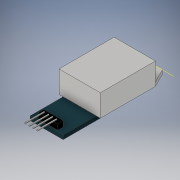
# Autodesk Inventor part: DHT22
Saved by Autodesk Inventor 2017.2 (Build 212223000, 223)
## iProperties
Created: 2017-03-02
Part Number: DHT22
Material: Generic
Document SubType Name: Modeling
Designer: prosp
Density: 1 g/cm^3
Appearance: Default
Author: prosp
Autodesk Inventor part; units mm, degrees
ref_plane "YZ Plane" through (0, 0, 0) normal (1, 0, 0) x (0, 1, 0)
ref_plane "XZ Plane" through (0, 0, 0) normal (0, 1, 0) x (-1, 0, 0)
ref_plane "XY Plane" through (0, 0, 0) normal (0, 0, 1) x (1, 0, 0)
sketch "Sketch1" plane through (0, 0, 0) normal (0, 1, 0) x (-1, 0, 0)
  line L0 (6, 14) -> (6, -14)
  line L1 (6, -14) -> (-6, -14)
  line L2 (-6, -14) -> (-6, 14)
  line L3 (-6, 14) -> (6, 14)
  line L4 (6, 14) -> (-6, -14) construction
  line L5 (6, -14) -> (-6, 14) construction
  line L6 (35.8902, -6.311) -> (20.8902, -6.311)
  line L7 (35.8902, -6.311) -> (35.8902, -26.311)
  line L8 (20.8902, -6.311) -> (20.8902, -26.311)
  line L9 (20.8902, -26.311) -> (23.3902, -31.311)
  line L10 (35.8902, -26.311) -> (33.3902, -31.311)
  line L11 (33.3902, -31.311) -> (23.3902, -31.311)
  point P0 (0, 0)
  dimension "d0" = 28
  dimension "d1" = 12
  dimension "d3" = 15
  dimension "d4" = 20
  dimension "d5" = 20
  constraints: 24 end point, 3 vertical, 2 horizontal, 2 midpoint, 2 parallel, 1 perpendicular, 1 point on line
  measures "d0" distance of L0.start L0.end
  measures "d1" distance of L0.end L1.end
  measures "d3" distance of L6.start L6.end
  measures "d4" distance of L6.start L7.end
  measures "d5" distance of L6.end L8.end
extrude "Extrusion1" add sketch "Sketch1" along normal blind 1.5 contours L0 L1 L2 L3
sketch "Sketch2" plane through (0, 1.5, 0) normal (0, 1, 0) x (1, 0, 0)
  line L0 (-6, -14) -> (6, -14) projected
  line L1 (-7.5, -2) -> (7.5, -2)
  line L2 (7.5, -2) -> (7.5, 18)
  line L3 (-7.5, 18) -> (-7.5, -2)
  line L4 (-7.5, 18) -> (-5, 23)
  line L5 (-5, 23) -> (5, 23)
  line L6 (5, 23) -> (7.5, 18)
  point P0 (0, 0)
  dimension "d14" = 15
  dimension "d15" = 20
  dimension "d16" = 15
  dimension "d19" = 10
  constraints: 12 end point, 2 horizontal, 1 vertical
  measures "d14" distance of L1.start L1.end
  measures "d15" distance of L1.end L2.end
  measures "d16" distance of L2.end L3.start
  measures "d19" distance of L4.end L5.end
extrude "Extrusion2" add sketch "Sketch2" along normal blind 1.5
sketch "Sketch3" plane through (0, 3, 0) normal (0, 1, 0) x (1, 0, 0)
  line L0 (-7.5, 18) -> (-7.5, -2) projected
  line L1 (7.5, -2) -> (7.5, 18) projected
  line L2 (-7.5, -2) -> (7.5, -2)
  line L3 (7.5, -2) -> (7.5, 18)
  line L4 (7.5, 18) -> (-7.5, 18)
  line L5 (-7.5, 18) -> (-7.5, -2)
  point P0 (0, 0)
  constraints: 8 end point, 2 parallel, 1 horizontal, 1 perpendicular
extrude "Extrusion3" add sketch "Sketch3" along normal blind 6.5
sketch "Sketch4" plane through (0, 1.5, 0) normal (0, 1, 0) x (1, 0, 0)
  line L0 (-6, -14) -> (6, -14) projected
  line L1 (-3.5, -13.5) -> (3.5, -13.5)
  line L2 (3.5, -13.5) -> (3.5, -11.5)
  line L3 (3.5, -11.5) -> (-3.5, -11.5)
  line L4 (-3.5, -11.5) -> (-3.5, -13.5)
  point P0 (0, 0)
  dimension "d27" = 7
  dimension "d28" = 2
  dimension "d29" = 7
  constraints: 8 end point, 1 perpendicular
  measures "d27" distance of L1.start L1.end
  measures "d28" distance of L1.end L2.end
  measures "d29" distance of L2.end L3.end
extrude "Extrusion4" add sketch "Sketch4" along normal blind 2
sketch "Sketch5" plane through (0, 3.5, 0) normal (0, 1, 0) x (1, 0, 0)
  point P0 (0, 0)
sketch "Sketch6" plane through (-3.5, 1.5, 13.5) normal (0, 0, 1) x (1, 0, 0)
  line L0 (0, 2) -> (7, 2) projected
  circle A0 centre (2.7375, 2.25) radius 0.25
  circle A1 centre (4.16, 2.25) radius 0.25
  circle A2 centre (5.6263, 2.25) radius 0.25
  circle A3 centre (1.1349, 2.25) radius 0.25
  point P0 (3.5, -1.5)
  dimension "d33" = 0.5
  dimension "d34" = 0.5
  dimension "d35" = 0.5
  dimension "d36" = 0.5
  constraints: 4 centre point, 1 tangent
  measures "d33" diameter of A0
  measures "d34" diameter of A1
  measures "d35" diameter of A2
  measures "d36" diameter of A3
extrude "Extrusion5" add sketch "Sketch6" along normal blind 6 and the other way blind 1
sketch "Sketch7" plane through (0, 3, 0) normal (0, 1, 0) x (1, 0, 0)
  line L0 (5, 23) -> (-5, 23) projected
  line L1 (-7.5, 18) -> (7.5, 18) projected
  line L2 (7.5, 18) -> (5, 23) projected
  line L3 (5, 23) -> (-5, 23) projected
  line L4 (-5, 23) -> (-7.5, 18) projected
  line L5 (-3.5, -13.5) -> (-3.5, -11.5) projected
  line L6 (-3.5, -11.5) -> (3.5, -11.5) projected
  line L7 (3.5, -11.5) -> (3.5, -13.5) projected
  line L8 (3.5, -13.5) -> (-3.5, -13.5) projected
  line L9 (-7.5, 18) -> (7.5, 18) projected
  line L10 (5, 23) -> (7.5, 18) projected
  line L11 (-5, 23) -> (5, 23) projected
  line L12 (-7.5, 18) -> (-5, 23) projected
  line L13 (-7.5, -2) -> (-7.5, 18) projected
  line L14 (7.5, -2) -> (-7.5, -2) projected
  line L15 (7.5, 18) -> (7.5, -2) projected
  circle A0 centre (0, 20) radius 1.5
  point P0 (0, 0)
  dimension "d44" = 3
  constraints: 1 centre point
  measures "d44" diameter of A0
hole "Hole1" at (0, 3, -20) direction (0, -1, 0) diameter 3 end through all
body "Solid1"
